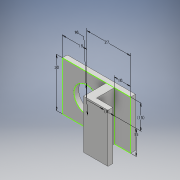
# Autodesk Inventor part: emswparts
Saved by Autodesk Inventor 2018.3 (Build 223284000, 284)
## iProperties
Created: 2019-12-20
Part Number: emswparts
Material: 一般
Document SubType Name: Modeling
Designer: Eiji Nishizawa
Density: 1 g/cm^3
Appearance: 既定
Author: Eiji Nishizawa
Autodesk Inventor part; units mm, degrees
ref_plane "YZ Plane" through (0, 0, 0) normal (1, 0, 0) x (0, 1, 0)
ref_plane "XZ Plane" through (0, 0, 0) normal (0, 1, 0) x (-1, 0, 0)
ref_plane "XY Plane" through (0, 0, 0) normal (0, 0, 1) x (1, 0, 0)
sketch "スケッチ1" plane through (0, 0, 0) normal (0, 1, 0) x (-1, 0, 0)
  line L0 (28.9798, 2.6849) -> (-13.0202, 2.6849)
  line L1 (-13.0202, 2.6849) -> (-13.0202, -27.3151)
  line L2 (-13.0202, -27.3151) -> (28.9798, -27.3151)
  line L3 (28.9798, -27.3151) -> (28.9798, 2.6849)
  circle A0 centre (13.9798, -12.3151) radius 8
  line L4 (-13.0202, 2.6849) -> (-3.0202, 2.6849)
  line L5 (-3.0202, 2.6849) -> (-3.0202, -27.3151)
  line L6 (-3.0202, -27.3151) -> (-13.0202, -27.3151)
  line L7 (-13.0202, -27.3151) -> (-13.0202, 2.6849)
  point P0 (0, 0)
  dimension "d0" = 16
  dimension "d1" = 30
  dimension "d2" = 15
  dimension "d3" = 15
  dimension "d4" = 15
  dimension "d5" = 27
  dimension "d6" = 10
  dimension "d7" = 9
  constraints: 16 end point, 4 parallel, 2 horizontal, 2 perpendicular, 1 centre point, 1 point on line
  measures "d0" diameter of A0
  measures "d1" distance of L2.end L0.start
  measures "d2" distance from line of L2 A0.centre
  measures "d3" distance from line of L0 A0.centre
  measures "d4" distance from line of L3 A0.centre
  measures "d5" distance from line of L1 A0.centre
  measures "d6" distance between parallel lines of L1 L5
  measures "d7" distance edge to line of A0 L5
extrude "押し出し1" add sketch "スケッチ1" along normal blind 3
sketch "スケッチ2" plane through (0, 0, 0) normal (0, -1, 0) x (1, 0, 0)
  line L0 (-28.9798, 2.6849) -> (13.0202, 2.6849) projected
  line L1 (13.0202, -27.3151) -> (-28.9798, -27.3151) projected
  line L2 (3.0499, 2.6849) -> (-1.9798, 2.6849)
  line L3 (-1.9798, 2.6849) -> (-1.9798, -27.3151)
  line L4 (-1.9798, -27.3151) -> (3.0499, -27.3151)
  line L5 (3.0499, -27.3151) -> (3.0499, 2.6849)
  circle A0 centre (-13.9798, -12.3151) radius 8 projected
  point P0 (0, 0)
  dimension "d10" = 4
  constraints: 8 end point, 2 parallel, 2 point on line, 1 horizontal, 1 perpendicular
  measures "d10" distance edge to line of A0 L3
extrude "押し出し2" add sketch "スケッチ2" along normal blind 14 contours L0 L5 L1 L3
sketch "スケッチ3" plane through (3.0499, 0, 2.6849) normal (1, 0, 0) x (0, 0, -1)
  line L0 (0, -14) -> (30, -14) projected
  line L1 (30, -14) -> (0, -14)
  line L2 (0, -14) -> (0, -11)
  line L3 (0, -11) -> (30, -11)
  line L4 (30, -11) -> (30, -14)
  line L5 (0, 0) -> (30, 0) projected
  point P0 (2.6849, 0)
  dimension "d13" = 3
  dimension "d14" = 11
  constraints: 8 end point, 2 parallel, 1 horizontal, 1 perpendicular
  measures "d13" distance of L1.end L2.end
  measures "d14" distance between parallel lines of L5 L3
extrude "押し出し3" add sketch "スケッチ3" along normal blind 10
